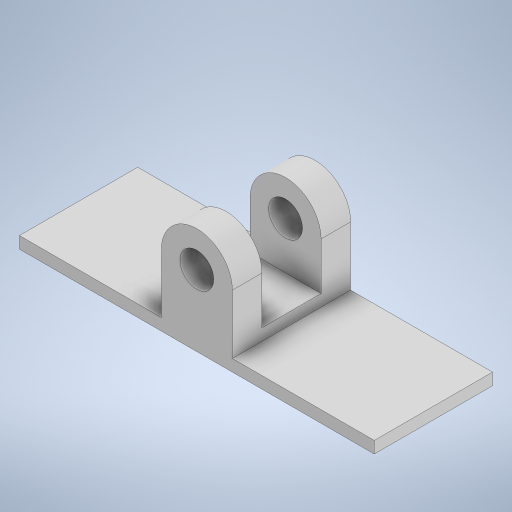
# Autodesk Inventor part: FingerTip
Saved by Autodesk Inventor 2023 (Build 270158000, 158)
## iProperties
Created: 2022-10-10
Part Number: FingerTip
Material: Generic
Document SubType Name: Modeling
Designer: GROS
Density: 1 g/cm^3
Appearance: Default
Author: GROS
Autodesk Inventor part; units mm, degrees
ref_plane "YZ Plane" through (0, 0, 0) normal (1, 0, 0) x (0, 1, 0)
ref_plane "XZ Plane" through (0, 0, 0) normal (0, 1, 0) x (-1, 0, 0)
ref_plane "XY Plane" through (0, 0, 0) normal (0, 0, 1) x (1, 0, 0)
sketch "Sketch1" plane through (0, 0, 0) normal (0, 1, 0) x (-1, 0, 0)
  line L0 (0, 0) -> (30, 0)
  line L1 (30, 0) -> (30, -10)
  line L2 (30, -10) -> (0, -10)
  line L3 (0, -10) -> (0, 0)
  dimension "d0" = 10
  dimension "d1" = 30
  constraints: 8 end point, 2 parallel, 1 horizontal, 1 perpendicular
  measures "d0" distance of L0.end L1.end
  measures "d1" distance of L1.end L2.end
extrude "Extrusion1" add sketch "Sketch1" along normal blind 1
sketch "Sketch2" plane through (0, 1, 0) normal (0, 1, 0) x (1, 0, 0)
  line L0 (-30, 10) -> (-30, 0) projected
  line L1 (-30, 5) -> (-15, 5)
  line L2 (-15, 5) -> (-15, 2.5)
  line L3 (-15, 2.5) -> (-18, 2.5)
  line L4 (-18, 2.5) -> (-12, 2.5)
  line L5 (-12, 2.5) -> (-12, 0)
  line L6 (-12, 0) -> (-18, 0)
  line L7 (-18, 0) -> (-18, 2.5)
  line L8 (-15, 5) -> (-15, 7.5)
  line L9 (-15, 7.5) -> (-18, 7.5)
  line L10 (-18, 7.5) -> (-12, 7.5)
  line L11 (-12, 7.5) -> (-12, 10)
  line L12 (-12, 10) -> (-18, 10)
  line L13 (-18, 10) -> (-18, 7.5)
  point P0 (0, 0)
  dimension "d4" = 15
  dimension "d5" = 2.5
  dimension "d20" = 3
  dimension "d21" = 2.5
  dimension "d22" = 6
  dimension "d23" = 2.5
  dimension "d24" = 3
  dimension "d25" = 2.5
  dimension "d26" = 6
  constraints: 26 end point, 4 horizontal, 4 parallel, 3 perpendicular, 2 vertical, 1 midpoint
  measures "d4" distance of L1.start L1.end
  measures "d5" distance of L1.end L2.end
  measures "d20" distance of L2.end L3.end
  measures "d21" distance of L6.end L3.end
  measures "d22" distance of L5.end L6.end
  measures "d23" distance of L1.end L8.end
  measures "d24" distance of L9.end L8.end
  measures "d25" distance of L12.end L9.end
  measures "d26" distance of L11.end L12.end
extrude "Extrusion2" add sketch "Sketch2" along normal blind 8
sketch "Sketch4" plane through (-30, 0, 0) normal (0, 0, 1) x (1, 0, 0)
  line L0 (12, 9) -> (18, 9) projected
  line L1 (15, 9) -> (15, 6)
  circle A0 centre (15, 6) radius 3
  circle A1 centre (15, 6) radius 1.425
  line L2 (18, 1) -> (18, 9) projected
  line L3 (12, 9) -> (18, 9)
  line L4 (18, 9) -> (18, 3)
  line L5 (18, 3) -> (12, 3)
  line L6 (12, 3) -> (12, 9)
  point P0 (30, 0)
  point P1 (12, 6)
  point P2 (18, 6)
  dimension "d27" = 3
  dimension "d28" = 2.85
  constraints: 10 end point, 2 coincident, 2 parallel, 1 centre point, 1 horizontal, 1 midpoint, 1 perpendicular, 1 point on line, 1 vertical, 3 other
  measures "d27" distance of L1.start L1.end
  measures "d28" diameter of A1
extrude "Extrusion4" cut sketch "Sketch4" against normal through all contours L0 A0 L6 | A1 | L0 L2 A0
sketch "Sketch5" plane through (0, 1, 0) normal (0, 1, 0) x (1, 0, 0)
  line L0 (-18, 2.5) -> (-18, 0) projected
  line L1 (-12, 7.5) -> (-18, 7.5) projected
  line L2 (-18, 2.5) -> (-12, 2.5)
  line L3 (-12, 2.5) -> (-12, 7.5)
  line L4 (-12, 7.5) -> (-18, 7.5)
  line L5 (-18, 7.5) -> (-18, 2.5)
  point P0 (0, 0)
  constraints: 8 end point, 2 parallel, 1 horizontal, 1 perpendicular
extrude "Extrusion5" add sketch "Sketch5" along normal blind 1
body "Solid1"
